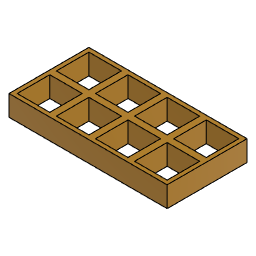
grid (Autodesk Fusion 360 design; units mm, degrees)
Autodesk Fusion 360 part; units mm, degrees
sketch "Sketch1" plane through (0, 0, 0) normal (0, 0, 1) x (1, 0, 0)
  line L0 (-84.8651, 33.3057) -> (-69.0651, 33.3057)
  line L1 (-69.0651, 33.3057) -> (-69.0651, 17.5057)
  line L2 (-69.0651, 17.5057) -> (-84.8651, 17.5057)
  line L3 (-84.8651, 17.5057) -> (-84.8651, 33.3057)
  line L4 (-84.8651, 33.3057) -> (-69.0651, 17.5057) construction
  line L5 (-69.0651, 33.3057) -> (-84.8651, 17.5057) construction
  line L6 (-50.0651, 33.3057) -> (-50.0651, 17.5057)
  line L7 (-65.8651, 33.3057) -> (-50.0651, 33.3057)
  line L8 (-65.8651, 17.5057) -> (-65.8651, 33.3057)
  line L9 (-50.0651, 17.5057) -> (-65.8651, 17.5057)
  line L10 (-31.0651, 33.3057) -> (-31.0651, 17.5057)
  line L11 (-46.8651, 33.3057) -> (-31.0651, 33.3057)
  line L12 (-46.8651, 17.5057) -> (-46.8651, 33.3057)
  line L13 (-31.0651, 17.5057) -> (-46.8651, 17.5057)
  line L14 (-12.0651, 33.3057) -> (-12.0651, 17.5057)
  line L15 (-27.8651, 33.3057) -> (-12.0651, 33.3057)
  line L16 (-27.8651, 17.5057) -> (-27.8651, 33.3057)
  line L17 (-12.0651, 17.5057) -> (-27.8651, 17.5057)
  line L18 (-69.0651, 52.3057) -> (-69.0651, 36.5057)
  line L19 (-84.8651, 52.3057) -> (-69.0651, 52.3057)
  line L20 (-84.8651, 36.5057) -> (-84.8651, 52.3057)
  line L21 (-69.0651, 36.5057) -> (-84.8651, 36.5057)
  line L22 (-50.0651, 52.3057) -> (-50.0651, 36.5057)
  line L23 (-65.8651, 52.3057) -> (-50.0651, 52.3057)
  line L24 (-65.8651, 36.5057) -> (-65.8651, 52.3057)
  line L25 (-50.0651, 36.5057) -> (-65.8651, 36.5057)
  line L26 (-31.0651, 52.3057) -> (-31.0651, 36.5057)
  line L27 (-46.8651, 52.3057) -> (-31.0651, 52.3057)
  line L28 (-46.8651, 36.5057) -> (-46.8651, 52.3057)
  line L29 (-31.0651, 36.5057) -> (-46.8651, 36.5057)
  line L30 (-12.0651, 52.3057) -> (-12.0651, 36.5057)
  line L31 (-27.8651, 52.3057) -> (-12.0651, 52.3057)
  line L32 (-27.8651, 36.5057) -> (-27.8651, 52.3057)
  line L33 (-12.0651, 36.5057) -> (-27.8651, 36.5057)
  line L34 (-86.8651, 54.3057) -> (-10.0651, 54.3057)
  line L35 (-10.0651, 54.3057) -> (-10.0651, 15.5057)
  line L36 (-10.0651, 15.5057) -> (-86.8651, 15.5057)
  line L37 (-86.8651, 15.5057) -> (-86.8651, 54.3057)
  point P0 (-76.9651, 25.4057)
  dimension "d3" = 15.8
  dimension "d4" = 15.8
  dimension "d7" = 19
  dimension "d8" = 19
  dimension "d9" = 2
  dimension "d10" = 2
  dimension "d11" = 2
  dimension "d12" = 2
  constraint horizontal L0
  constraint perpendicular L0 L1
  constraint parallel L0 L2
  constraint parallel L1 L3
  constraint coincident L4 P0
  constraint coincident L5 P0
  constraint horizontal L34
  constraint vertical L35
  constraint horizontal L36
  constraint vertical L37
  measures "d3" distance of L0 L2
  measures "d4" distance of L1 L3
  measures "d9" distance of L20 L37
  measures "d10" distance of L23 L34
  measures "d11" distance of L30 L35
  measures "d12" distance of L13 L36
extrude "Extrude1" add sketch "Sketch1" along normal blind 10
